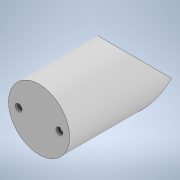
# Autodesk Inventor part: 20220524_吸引部分筒
Saved by Autodesk Inventor 2020 (Build 240168000, 168)
## iProperties
Created: 2022-05-22
Part Number: 20220524_吸引部分筒
Material: 一般
Document SubType Name: Modeling
Designer: Naggy
Density: 1 g/cm^3
Appearance: 既定
Author: Naggy
Autodesk Inventor part; units mm, degrees
ref_plane "YZ Plane" through (0, 0, 0) normal (1, 0, 0) x (0, 1, 0)
ref_plane "XZ Plane" through (0, 0, 0) normal (0, 1, 0) x (-1, 0, 0)
ref_plane "XY Plane" through (0, 0, 0) normal (0, 0, 1) x (1, 0, 0)
sketch "スケッチ1" plane through (0, 0, 0) normal (0, 0, 1) x (1, 0, 0)
  circle A0 centre (0, 0) radius 15
  dimension "d0" = 30
  constraints: 1 centre point, 1 coincident
  measures "d0" diameter of A0
extrude "押し出し1" add sketch "スケッチ1" along normal blind 30
sketch "スケッチ2" plane through (0, 0, 30) normal (0, 0, 1) x (1, 0, 0)
  circle A0 centre (0, 0) radius 15
  dimension "d3" = 30
  constraints: 1 centre point, 1 coincident
  measures "d3" diameter of A0
extrude "押し出し2" add sketch "スケッチ2" along normal blind 20
sketch "スケッチ4" plane through (0, 0, 0) normal (1, 0, 0) x (0, 1, 0)
  point P0 (0, 0)
sketch "スケッチ5" plane through (0, 0, 0) normal (0, 0, -1) x (-1, 0, 0)
  circle A0 centre (0, 0) radius 14
  dimension "d6" = 28
  constraints: 1 centre point, 1 coincident
  measures "d6" diameter of A0
extrude "押し出し3" cut sketch "スケッチ5" against normal blind 48
sketch "スケッチ6" plane through (0, 0, 0) normal (0, 1, 0) x (-1, 0, 0)
  line L0 (15, 0) -> (-15, 0) projected
  arc A0 (15, 0) -> (-15, 0) centre (0, 0) ccw
  constraints: 2 point on circle, 1 centre point, 1 coincident
extrude "押し出し4" cut sketch "スケッチ6" along normal blind 50 and the other way blind 25
sketch "スケッチ7" plane through (0, 0, 50) normal (0, 0, 1) x (1, 0, 0)
  point P0 (0, 0)
  point P1 (10, 0)
  point P2 (-10, 0)
  dimension "d14" = 10
  dimension "d15" = 10
  measures "d14" distance of point (10, 0) point (0, 0)
  measures "d15" distance of point (-10, 0) point (0, 0)
hole "穴1" at (10, 0, 50) at (-10, 0, 50) direction (0, 0, -1) diameter 3.4 end through all clearance for "Flat Head Machine Screw" size "M3" standard "Ansi Metric M Profile"
